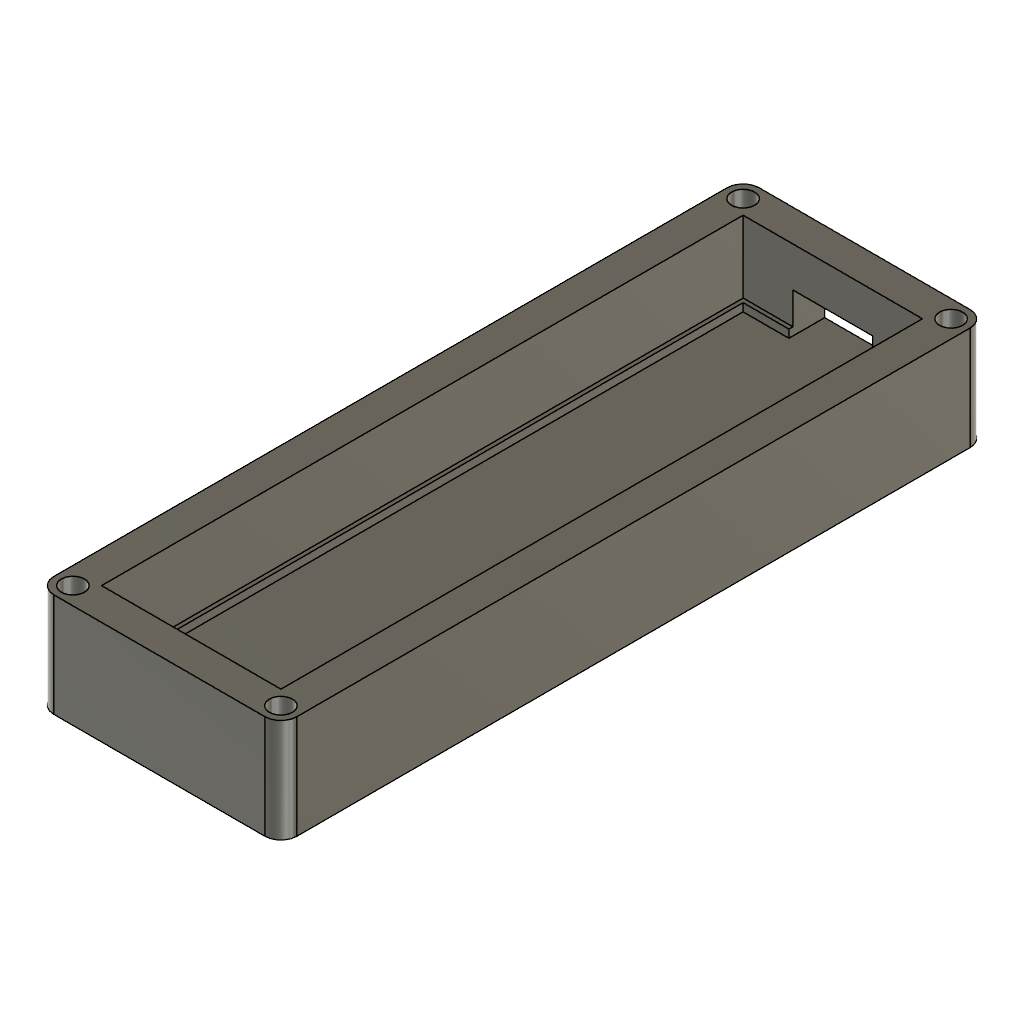
macropad (Autodesk Fusion 360 design; units mm, degrees)
part number: 2026-09-19-16-12-25-873
Autodesk Fusion 360 part; units mm, degrees
sketch "Sketch1" plane through (0, 0, 0) normal (0, 0, 1) x (1, 0, 0)
  line L0 (0, 0) -> (22.5, 0)
  line L1 (22.5, 0) -> (22.5, 80.5)
  line L2 (22.5, 80.5) -> (0, 80.5)
  line L3 (0, 80.5) -> (0, 0)
  dimension "d1" = 22.5
  dimension "d2" = 80.5
  constraint horizontal L0
  constraint vertical L1
  constraint horizontal L2
  constraint vertical L3
  constraint coincident L0.start L3.end
  measures "d1" distance of L0.start L0.end
  measures "d2" distance of L0.start L2.end
extrude "Extrude1" add sketch "Sketch1" along normal blind 1
sketch "Sketch2" plane through (0, 0, 0) normal (0, 0, 1) x (1, 0, 0)
  line L0 (0, -3) -> (22.5, -3)
  line L1 (22.5, -3) -> (25.5, -3)
  line L2 (25.5, -3) -> (25.5, 0)
  line L3 (0, 0) -> (-3, 0)
  line L4 (-3, 0) -> (-3, -3)
  line L5 (-3, -3) -> (0, -3)
  line L6 (-3, 0) -> (-3, 80.5)
  line L7 (-3, 80.5) -> (-3, 83.5)
  line L8 (-3, 83.5) -> (0, 83.5)
  line L9 (0, 83.5) -> (22.5, 83.5)
  line L10 (22.5, 80.5) -> (0, 80.5)
  line L11 (0, 80.5) -> (0, 0)
  line L12 (22.5, 83.5) -> (25.5, 83.5)
  line L13 (25.5, 83.5) -> (25.5, 80.5)
  line L14 (25.5, 80.5) -> (25.5, 0)
  line L15 (0, 0) -> (22.5, 0)
  line L16 (22.5, 0) -> (22.5, 80.5)
  line L17 (0, 80.5) -> (22.5, 80.5)
  line L18 (0, 80.5) -> (0, 0)
  constraint coincident L3.start L11.end
  constraint perpendicular L1 L2
  constraint perpendicular L3 L4
  constraint perpendicular L6 L8
  constraint perpendicular L6 L9
  constraint perpendicular L3 L11
  constraint perpendicular L9 L13
  constraint perpendicular L11 L15
extrude "Extrude2" add sketch "Sketch2" along normal blind 5
extrude "Extrude3" add 1 faces at (7.5, 53.6667, 1) along direction (0, 0, 1) blind 2
extrude "Extrude4" add 1 faces at (-2, 53.6667, 5) along direction (0, 0, 1) blind 8
sketch "Sketch3" plane through (0, 0, 3) normal (0, 0, 1) x (-1, 0, 0)
  line L0 (0, -80.5) -> (0, 0)
  line L1 (0, 0) -> (-22.5, 0)
  line L2 (-22.5, 0) -> (-22.5, -80.5)
  line L3 (-22.5, -80.5) -> (0, -80.5)
  line L4 (-22, -0.5) -> (-0.5, -0.5)
  line L5 (-0.5, -0.5) -> (-0.5, -80)
  line L6 (-0.5, -80) -> (-22, -80)
  line L7 (-22, -80) -> (-22, -0.5)
  constraint horizontal L4
  constraint vertical L5
  constraint horizontal L6
  constraint vertical L7
extrude "Extrude5" add sketch "Sketch3" along normal blind 1
sketch "Sketch4" plane through (0, 0, 0) normal (0, 0, 1) x (1, 0, 0)
  line L0 (-3, -4) -> (-4, -4)
  line L1 (-4, -4) -> (-4, -3)
  line L2 (-3, -4) -> (25.5, -4)
  line L3 (25.5, -4) -> (26.5, -4)
  line L4 (26.5, -4) -> (26.5, -3)
  line L5 (26.5, -3) -> (26.5, 83.5)
  line L6 (26.5, 83.5) -> (26.5, 84.5)
  line L7 (26.5, 84.5) -> (25.5, 84.5)
  line L8 (25.5, 84.5) -> (-3, 84.5)
  line L9 (-3, 84.5) -> (-4, 84.5)
  line L10 (-4, 84.5) -> (-4, 83.5)
  line L11 (-4, 83.5) -> (-4, 84.5)
  line L12 (-4, 83.5) -> (-4, -3)
  line L13 (-3, 84.5) -> (-4, 84.5)
  line L14 (-4, 84.5) -> (-4, -4)
  line L15 (-4, -4) -> (26.5, -4)
  line L16 (26.5, -4) -> (26.5, 84.5)
  line L17 (26.5, -4) -> (26.5, 84.5)
  line L18 (26.5, 84.5) -> (-4, 84.5)
  line L19 (-4, 84.5) -> (-4, -4)
  line L20 (-4, -3) -> (-4, -4)
  line L21 (-4, -4) -> (26.5, -4)
  line L22 (25.5, 83.5) -> (-3, 83.5)
  line L23 (-3, 83.5) -> (-3, -3)
  line L24 (-3, -3) -> (25.5, -3)
  line L25 (25.5, -3) -> (25.5, 83.5)
  constraint perpendicular L0 L1
  constraint perpendicular L3 L4
  constraint perpendicular L2 L5
  constraint perpendicular L2 L6
  constraint perpendicular L5 L7
  constraint perpendicular L9 L10
  constraint perpendicular L0 L14
  constraint perpendicular L4 L15
  constraint perpendicular L7 L16
  constraint perpendicular L12 L22
  constraint perpendicular L21 L23
  constraint perpendicular L23 L24
  constraint perpendicular L22 L25
extrude "Extrude6" add sketch "Sketch4" along normal blind 13
sketch "Sketch5" plane through (0, 0, 13) normal (0, 0, 1) x (-1, 0, 0)
  line L0 (4, 4) -> (-26.5, 4)
  line L1 (-26.5, 4) -> (-26.5, -84.5)
  line L2 (-26.5, -84.5) -> (4, -84.5)
  line L3 (4, -84.5) -> (4, 4)
  line L4 (0, 0) -> (0, -80.5)
  line L5 (0, -80.5) -> (-22.5, -80.5)
  line L6 (-22.5, -80.5) -> (-22.5, 0)
  line L7 (-22.5, 0) -> (0, 0)
  line L8 (0, 0) -> (1.5, 0)
  line L9 (1.5, 0) -> (1.8, 0)
  line L10 (1.8, 0) -> (1.8, 1.8)
  dimension "d15" = 1.8
  constraint coincident L4.start L7.end
  constraint perpendicular L4 L8
  constraint perpendicular L4 L9
  constraint perpendicular L9 L10
  measures "d15" distance of L9.end L10.end
hole "Hole1" at (-1.8, -1.8, 13) direction (0, 0, -1) diameter 2.9 depth 13 tip angle 118
sketch "Sketch6" plane through (0, 0, 13) normal (0, 0, 1) x (-1, 0, 0)
  circle A0 centre (1.8, 1.8) radius 1.45
  line L0 (4, 4) -> (-26.5, 4)
  line L1 (-26.5, 4) -> (-26.5, -84.5)
  line L2 (-26.5, -84.5) -> (4, -84.5)
  line L3 (4, -84.5) -> (4, 4)
  line L4 (0, 0) -> (0, -80.5)
  line L5 (0, -80.5) -> (-22.5, -80.5)
  line L6 (-22.5, -80.5) -> (-22.5, 0)
  line L7 (-22.5, 0) -> (0, 0)
  line L8 (-22.5, 0) -> (-22.5, 1.8)
  line L9 (-22.5, 1.8) -> (-24.3, 1.8)
  dimension "d19" = 1.8
  dimension "d20" = 1.8
  constraint coincident L6.end L7.start
  constraint perpendicular L7 L8
  constraint perpendicular L8 L9
  measures "d19" distance of L6.end L8.end
  measures "d20" distance of L8.end L9.end
hole "Hole2" at (24.3, -1.8, 13) direction (0, 0, -1) diameter 2.9 depth 13 tip angle 118
sketch "Sketch7" plane through (0, 0, 13) normal (0, 0, 1) x (-1, 0, 0)
  circle A0 centre (-24.3, 1.8) radius 1.45
  circle A1 centre (1.8, 1.8) radius 1.45
  line L0 (4, 4) -> (-26.5, 4)
  line L1 (-26.5, 4) -> (-26.5, -84.5)
  line L2 (-26.5, -84.5) -> (4, -84.5)
  line L3 (4, -84.5) -> (4, 4)
  line L4 (0, 0) -> (0, -80.5)
  line L5 (0, -80.5) -> (-22.5, -80.5)
  line L6 (-22.5, -80.5) -> (-22.5, 0)
  line L7 (-22.5, 0) -> (0, 0)
  line L8 (0, -80.5) -> (0, -82.3)
  line L9 (0, -82.3) -> (1.8, -82.3)
  dimension "d24" = 1.8
  dimension "d25" = 1.8
  constraint coincident L4.end L5.start
  constraint perpendicular L5 L8
  constraint perpendicular L8 L9
  measures "d24" distance of L4.end L8.end
  measures "d25" distance of L8.end L9.end
hole "Hole3" at (-1.8, 82.3, 13) direction (0, 0, -1) diameter 2.9 depth 13 tip angle 118
sketch "Sketch8" plane through (0, 0, 13) normal (0, 0, 1) x (-1, 0, 0)
  circle A0 centre (1.8, -82.3) radius 1.45
  circle A1 centre (-24.3, 1.8) radius 1.45
  circle A2 centre (1.8, 1.8) radius 1.45
  line L0 (4, 4) -> (-26.5, 4)
  line L1 (-26.5, 4) -> (-26.5, -84.5)
  line L2 (-26.5, -84.5) -> (4, -84.5)
  line L3 (4, -84.5) -> (4, 4)
  line L4 (0, 0) -> (0, -80.5)
  line L5 (0, -80.5) -> (-22.5, -80.5)
  line L6 (-22.5, -80.5) -> (-22.5, 0)
  line L7 (-22.5, 0) -> (0, 0)
  line L8 (-22.5, -80.5) -> (-24.3, -80.5)
  line L9 (-24.3, -80.5) -> (-24.3, -82.3)
  dimension "d29" = 1.8
  dimension "d30" = 1.8
  constraint coincident L5.end L6.start
  constraint perpendicular L6 L8
  constraint perpendicular L8 L9
  measures "d29" distance of L5.end L8.end
  measures "d30" distance of L8.end L9.end
hole "Hole4" at (24.3, 82.3, 13) direction (0, 0, -1) diameter 2.9 depth 13 tip angle 118
sketch "Sketch9" plane through (0, 0, 13) normal (0, 0, 1) x (-1, 0, 0)
  circle A0 centre (-24.3, -82.3) radius 1.45
  circle A1 centre (1.8, -82.3) radius 1.45
  circle A2 centre (-24.3, 1.8) radius 1.45
  circle A3 centre (1.8, 1.8) radius 1.45
  line L0 (4, 4) -> (-26.5, 4)
  line L1 (-26.5, 4) -> (-26.5, -84.5)
  line L2 (-26.5, -84.5) -> (4, -84.5)
  line L3 (4, -84.5) -> (4, 4)
  line L4 (0, 0) -> (0, -80.5)
  line L5 (0, -80.5) -> (-22.5, -80.5)
  line L6 (-22.5, -80.5) -> (-22.5, 0)
  line L7 (-22.5, 0) -> (0, 0)
  line L8 (2, 4) -> (-26.5, 4)
  line L9 (-26.5, 4) -> (-26.5, -84.5)
  line L10 (-26.5, -84.5) -> (4, -84.5)
  line L11 (4, -84.5) -> (4, 2)
  arc A4 (4, 2) -> (2, 4) centre (2, 2) ccw
  dimension "d34" = 2
  constraint coincident L0.end L1.start
  constraint coincident L1.end L2.start
  constraint coincident L2.end L3.start
  constraint tangent L8 A4
  constraint tangent L11 A4
  measures "d34" radius of A4
extrude "Extrude7" cut sketch "Sketch9" against normal blind 13 contours L0 L3 A4
sketch "Sketch10" plane through (0, 0, 13) normal (0, 0, 1) x (-1, 0, 0)
  arc A0 (4, 2) -> (2, 4) centre (2, 2) ccw
  line L0 (2, 4) -> (-26.5, 4)
  line L1 (-26.5, 4) -> (-26.5, -84.5)
  line L2 (-26.5, -84.5) -> (4, -84.5)
  line L3 (4, -84.5) -> (4, 2)
  circle A1 centre (-24.3, -82.3) radius 1.45
  circle A2 centre (1.8, -82.3) radius 1.45
  circle A3 centre (-24.3, 1.8) radius 1.45
  circle A4 centre (1.8, 1.8) radius 1.45
  line L4 (0, 0) -> (0, -80.5)
  line L5 (0, -80.5) -> (-22.5, -80.5)
  line L6 (-22.5, -80.5) -> (-22.5, 0)
  line L7 (-22.5, 0) -> (0, 0)
  line L8 (2, -84.5) -> (-26.5, -84.5)
  line L9 (4, -82.5) -> (4, -67)
  arc A5 (2, -84.5) -> (4, -82.5) centre (2, -82.5) ccw
  dimension "d37" = 2
  constraint coincident L1.end L2.start
  constraint coincident L3 L9.end
  constraint tangent L9 A5
  constraint tangent L8 A5
  measures "d37" radius of A5
extrude "Extrude8" cut sketch "Sketch10" against normal blind 13 contours L2 L3 A5
sketch "Sketch11" plane through (0, 0, 13) normal (0, 0, 1) x (-1, 0, 0)
  line L0 (0, 0) -> (0, -80.5)
  line L1 (0, -80.5) -> (-22.5, -80.5)
  line L2 (-22.5, -80.5) -> (-22.5, 0)
  line L3 (-22.5, 0) -> (0, 0)
  circle A0 centre (1.8, 1.8) radius 1.45
  circle A1 centre (-24.3, 1.8) radius 1.45
  circle A2 centre (1.8, -82.3) radius 1.45
  circle A3 centre (-24.3, -82.3) radius 1.45
  arc A4 (2, -84.5) -> (4, -82.5) centre (2, -82.5) ccw
  line L4 (4, -82.5) -> (4, 2)
  arc A5 (4, 2) -> (2, 4) centre (2, 2) ccw
  line L5 (2, 4) -> (-26.5, 4)
  line L6 (-26.5, 4) -> (-26.5, -84.5)
  line L7 (-26.5, -84.5) -> (2, -84.5)
  line L8 (-17, 4) -> (-24.5, 4)
  line L9 (-26.5, -5.3721) -> (-26.5, 2)
  arc A6 (-24.5, 4) -> (-26.5, 2) centre (-24.5, 2) ccw
  dimension "d40" = 2
  constraint coincident L5 L8.start
  constraint coincident L6 L9.start
  constraint tangent L8 A6
  constraint tangent L9 A6
  measures "d40" radius of A6
extrude "Extrude9" cut sketch "Sketch11" against normal blind 13 contours L5 L6 A6
sketch "Sketch12" plane through (0, 0, 13) normal (0, 0, 1) x (-1, 0, 0)
  arc A0 (-24.5, 4) -> (-26.5, 2) centre (-24.5, 2) ccw
  line L0 (-26.5, 2) -> (-26.5, -84.5)
  line L1 (-26.5, -84.5) -> (2, -84.5)
  arc A1 (2, -84.5) -> (4, -82.5) centre (2, -82.5) ccw
  line L2 (4, -82.5) -> (4, 2)
  arc A2 (4, 2) -> (2, 4) centre (2, 2) ccw
  line L3 (2, 4) -> (-24.5, 4)
  line L4 (0, 0) -> (0, -80.5)
  line L5 (0, -80.5) -> (-22.5, -80.5)
  line L6 (-22.5, -80.5) -> (-22.5, 0)
  line L7 (-22.5, 0) -> (0, 0)
  circle A3 centre (1.8, 1.8) radius 1.45
  circle A4 centre (-24.3, 1.8) radius 1.45
  circle A5 centre (1.8, -82.3) radius 1.45
  circle A6 centre (-24.3, -82.3) radius 1.45
  line L8 (-26.5, -80.5) -> (-26.5, -82.5)
  line L9 (-19.8373, -84.5) -> (-24.5, -84.5)
  arc A7 (-26.5, -82.5) -> (-24.5, -84.5) centre (-24.5, -82.5) ccw
  dimension "d43" = 2
  constraint coincident L0 L8.start
  constraint coincident L1 L9.start
  constraint tangent L8 A7
  constraint tangent L9 A7
  measures "d43" radius of A7
extrude "Extrude10" cut sketch "Sketch12" against normal blind 13 contours L0 L1 A7
sketch "Sketch13" plane through (0, 84.5, 0) normal (0, 1, 0) x (-1, 0, 0)
  line L0 (-24.5, 13) -> (-24.5, 0)
  line L1 (-24.5, 0) -> (2, 0)
  line L2 (2, 0) -> (2, 13)
  line L3 (2, 13) -> (-24.5, 13)
  line L4 (-24.5, 13) -> (-11.25, 13)
  line L5 (-11.25, 13) -> (-16.25, 13)
  line L6 (-11.25, 13) -> (-6.25, 13)
  line L7 (-16.25, 13) -> (-16.25, 8)
  line L8 (-16.25, 8) -> (-6, 8)
  line L9 (-6.25, 13) -> (-6.25, 8)
  line L10 (-16.25, 8) -> (-16.25, 3)
  line L11 (-16.25, 3) -> (-6.25, 3)
  line L12 (-6.25, 3) -> (-6.25, 8)
  dimension "d46" = 13.25
  dimension "d47" = 5
  dimension "d48" = 5
  constraint coincident L0.start L3.end
  constraint perpendicular L2 L4
  constraint parallel L3 L5
  constraint parallel L3 L6
  constraint perpendicular L1 L7
  constraint perpendicular L7 L8
  constraint coincident L8 L9.end
  constraint perpendicular L8 L9
  constraint perpendicular L8 L10
  constraint perpendicular L10 L11
  constraint perpendicular L8 L12
  measures "d46" distance of L0.start L4.end
  measures "d47" distance of L4.end L5.end
  measures "d48" distance of L4.end L6.end
extrude "Extrude11" cut sketch "Sketch13" against normal blind 5 contours L8 L10 L11 L12
